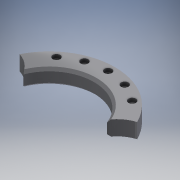
# Autodesk Inventor part: Funnel_Adapter
Saved by Autodesk Inventor 2016 (Build 200138000, 138)
## iProperties
Created: 2015-07-20
Part Number: Funnel_Adapter
Material: Generic
Document SubType Name: Modeling
Designer: bastli
Density: 1 g/cm^3
Appearance: Default
Author: bastli
Autodesk Inventor part; units mm, degrees
ref_plane "YZ Plane" through (0, 0, 0) normal (1, 0, 0) x (0, 1, 0)
ref_plane "XZ Plane" through (0, 0, 0) normal (0, 1, 0) x (-1, 0, 0)
ref_plane "XY Plane" through (0, 0, 0) normal (0, 0, 1) x (1, 0, 0)
derived "Transmission.ipt"
sketch "Sketch1" plane through (0, 0, 0) normal (0, 0, 1) x (1, 0, 0)
  circle A0 centre (-40.963, -23.65) radius 1.55 construction
  circle A1 centre (-30.4039, -36.2339) radius 1.55 construction
  circle A2 centre (-21.0753, -57.9039) radius 1.55 construction
  circle A3 centre (0, -47.3) radius 1.55 construction
  circle A4 centre (16.1776, -44.4475) radius 1.55 construction
  circle A5 centre (39.6086, -47.2037) radius 1.55 construction
  circle A6 centre (40.963, -23.65) radius 1.55 construction
  circle A7 centre (-40.963, 23.65) radius 1.55 construction
  circle A8 centre (-30.4039, 36.2339) radius 1.55 construction
  circle A9 centre (-16.1776, 44.4475) radius 1.55 construction
  circle A10 centre (53.3645, 30.81) radius 1.55 construction
  circle A11 centre (39.6086, 47.2037) radius 1.55 construction
  circle A12 centre (21.0753, 57.9039) radius 1.55 construction
  circle A13 centre (0, 61.62) radius 1.55 construction
  circle A14 centre (0, 47.3) radius 1.55 construction
  circle A15 centre (16.1776, 44.4475) radius 1.55 construction
  circle A16 centre (30.4039, 36.2339) radius 1.55 construction
  circle A17 centre (40.963, 23.65) radius 1.55 construction
  circle A18 centre (-21.0753, 57.9039) radius 1.55 construction
  circle A19 centre (-39.6086, 47.2037) radius 1.55 construction
  circle A20 centre (-53.3645, 30.81) radius 1.55 construction
  circle A21 centre (53.3645, -30.81) radius 1.55 construction
  circle A22 centre (30.4039, -36.2339) radius 1.55 construction
  circle A23 centre (21.0753, -57.9039) radius 1.55 construction
  circle A24 centre (0, -61.62) radius 1.55 construction
  circle A25 centre (-16.1776, -44.4475) radius 1.55 construction
  circle A26 centre (-39.6086, -47.2037) radius 1.55 construction
  circle A27 centre (-53.3645, -30.81) radius 1.55 construction
  circle A28 centre (62.46, 8) radius 2.2 construction
  circle A29 centre (46.46, -8) radius 2.2 construction
  circle A30 centre (-46.46, -8) radius 2.2 construction
  circle A31 centre (-62.46, 8) radius 2.2 construction
  circle A32 centre (-46.46, 8) radius 2.2 construction
  circle A33 centre (-62.46, -8) radius 2.2 construction
  circle A34 centre (46.46, 8) radius 2.2 construction
  circle A35 centre (62.46, -8) radius 2.2 construction
  circle A36 centre (-54.46, 0) radius 7.995 construction
  circle A37 centre (54.46, 0) radius 7.995 construction
  circle A38 centre (0, 0) radius 37.3 construction
  circle A39 centre (0.1505, 0.0441) radius 36 construction
  circle A40 centre (-54.46, 0) radius 21.46 construction
  circle A41 centre (54.46, 0) radius 21.46 construction
  circle A42 centre (-54.46, 0) radius 24.46 construction
  circle A43 centre (54.46, 0) radius 24.46 construction
  circle A44 centre (0.1505, 0.0441) radius 52.4157 construction
  line L0 (0.1505, 37.2997) -> (0.1505, 52.4598) construction
  line L1 (0.1505, 52.4598) -> (0.1505, 67.6198) construction
  line L2 (0.1505, 0.0441) -> (0.1505, 37.2997) construction
  arc A45 (33.7393, 12.9978) -> (-33.553, 12.696) centre (0.1505, 0.0441) ccw
  circle A46 centre (54.61, 0) radius 2.1 projected
  arc A47 (47.0732, 23.4036) -> (33.7393, 12.9978) centre (54.61, 0) ccw
  arc A48 (47.0732, 23.4036) -> (-46.8502, 23.2461) centre (0.1505, 0.0441) ccw
  arc A49 (-33.553, 12.696) -> (-46.8502, 23.2461) centre (-54.46, 0) ccw
  arc A50 (5.7928, 67.3714) -> (-5.7928, 67.3714) centre (0, 0) ccw projected
  arc A51 (-61.2418, -28.669) -> (-65.342, -17.4038) centre (-63.542, -23.1274) ccw projected
  arc A52 (-61.2418, -28.669) -> (-55.4489, -38.7025) centre (0, 0) ccw projected
  arc A53 (-47.7431, -47.8859) -> (-55.4489, -38.7025) centre (-51.7999, -43.4653) ccw projected
  arc A54 (-47.7431, -47.8859) -> (-38.8679, -55.3331) centre (0, 0) ccw projected
  arc A55 (-28.4859, -61.3272) -> (-38.8679, -55.3331) centre (-33.81, -58.5606) ccw projected
  arc A56 (-28.4859, -61.3272) -> (-17.5989, -65.2897) centre (0, 0) ccw projected
  arc A57 (-5.7928, -67.3714) -> (-17.5989, -65.2897) centre (-11.7421, -66.5927) ccw projected
  arc A58 (-5.7928, -67.3714) -> (5.7928, -67.3714) centre (0, 0) ccw projected
  arc A59 (17.5989, -65.2897) -> (5.7928, -67.3714) centre (11.7421, -66.5927) ccw projected
  arc A60 (17.5989, -65.2897) -> (28.4859, -61.3272) centre (0, 0) ccw projected
  arc A61 (38.8679, -55.3331) -> (28.4859, -61.3272) centre (33.81, -58.5606) ccw projected
  arc A62 (38.8679, -55.3331) -> (47.7431, -47.8859) centre (0, 0) ccw projected
  arc A63 (55.4489, -38.7025) -> (47.7431, -47.8859) centre (51.7999, -43.4653) ccw projected
  arc A64 (55.4489, -38.7025) -> (61.2418, -28.669) centre (0, 0) ccw projected
  arc A65 (65.342, -17.4038) -> (61.2418, -28.669) centre (63.542, -23.1274) ccw projected
  arc A66 (65.342, -17.4038) -> (65.342, 17.4038) centre (0, 0) ccw projected
  arc A67 (61.2418, 28.669) -> (65.342, 17.4038) centre (63.542, 23.1274) ccw projected
  arc A68 (61.2418, 28.669) -> (55.4489, 38.7025) centre (0, 0) ccw projected
  arc A69 (47.7431, 47.8859) -> (55.4489, 38.7025) centre (51.7999, 43.4653) ccw projected
  arc A70 (28.4859, 61.3272) -> (38.8679, 55.3331) centre (33.81, 58.5606) ccw projected
  arc A71 (28.4859, 61.3272) -> (17.5989, 65.2897) centre (0, 0) ccw projected
  arc A72 (5.7928, 67.3714) -> (17.5989, 65.2897) centre (11.7421, 66.5927) ccw projected
  arc A73 (-17.5989, 65.2897) -> (-5.7928, 67.3714) centre (-11.7421, 66.5927) ccw projected
  arc A74 (-17.5989, 65.2897) -> (-28.4859, 61.3272) centre (0, 0) ccw projected
  arc A75 (-38.8679, 55.3331) -> (-28.4859, 61.3272) centre (-33.81, 58.5606) ccw projected
  arc A76 (-38.8679, 55.3331) -> (-47.7431, 47.8859) centre (0, 0) ccw projected
  arc A77 (-55.4489, 38.7025) -> (-47.7431, 47.8859) centre (-51.7999, 43.4653) ccw projected
  arc A78 (-55.4489, 38.7025) -> (-61.2418, 28.669) centre (0, 0) ccw projected
  arc A79 (-65.342, 17.4038) -> (-61.2418, 28.669) centre (-63.542, 23.1274) ccw projected
  arc A80 (-65.342, 17.4038) -> (-65.342, -17.4038) centre (0, 0) ccw projected
  arc A81 (47.7431, 47.8859) -> (38.8679, 55.3331) centre (0, 0) ccw projected
  point P0 (0, 0)
  dimension "d0" = 72
  dimension "d3" = 42.92
  dimension "d4" = 42.92
  dimension "d6" = 3
  dimension "d7" = 3
  constraints: 19 coincident, 11 point on circle, 7 centre point, 6 end point, 2 vertical, 1 collinear, 1 point on line, 11 other
  measures "d3" diameter of A40
  measures "d4" diameter of A41
extrude "Extrusion1" add sketch "Sketch1" along normal blind 12.7 contours A45 A49 A48 A47
sketch "Sketch2" plane through (0, 0, 12.7) normal (0, 0, 1) x (1, 0, 0)
  circle A0 centre (-30.4039, 36.2339) radius 1.55 projected
  circle A1 centre (-16.1776, 44.4475) radius 1.55 projected
  circle A2 centre (0, 47.3) radius 1.55 projected
  circle A3 centre (16.1776, 44.4475) radius 1.55 projected
  circle A4 centre (30.4039, 36.2339) radius 1.55 projected
  point P0 (0, 0)
  constraints: 5 coincident
hole "Hole1" at (-30.4039, 36.2339, 12.7) at (0, 47.3, 12.7) at (30.4039, 36.2339, 12.7) at (16.1776, 44.4475, 12.7) at (-16.1776, 44.4475, 12.7) direction (0, 0, -1) diameter 3.1 end through all
hole "Hole2" at (-30.4039, 36.2339, 12.7) at (-16.1776, 44.4475, 12.7) at (0, 47.3, 12.7) at (16.1776, 44.4475, 12.7) at (30.4039, 36.2339, 12.7) direction (0, 0, -1) diameter 6 depth 3
chamfer "Chamfer1" distance 2 angle 45 1 edges at (-0.0109, 36.0437, 0)
chamfer "Chamfer2" distance 2 angle 45 1 edges at (-0.0109, 36.0437, 12.7)
equation "\"d0\" = funnel_width"
equation "\"d3\" = d5"
equation "\"d4\" = d5"
equation "\"d7\" = thickness"
equation "\"funnel_width\" = 72"
equation "\"thickness\" = 3"
equation "\"d5\" = 42.92"
body "Solid1"
